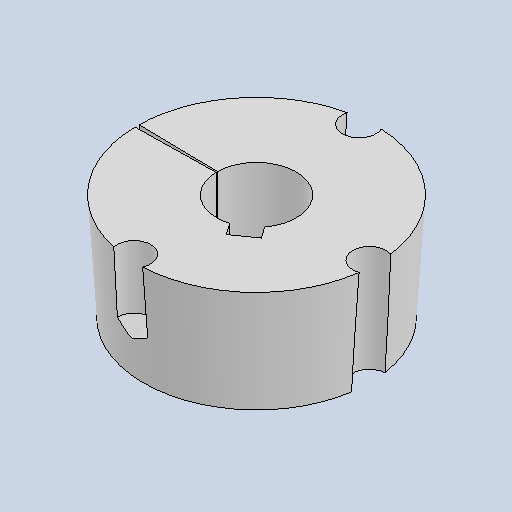
# Autodesk Inventor part: Втулка для шкива
Saved by Autodesk Inventor 2025 (Build 290162010, 162A)
## iProperties
Created: 2024-04-09
Part Number: Втулка для шкива
Material: Generic
Document SubType Name: Modeling
Designer: pokla
Density: 1 g/cm^3
Appearance: Default
Stock Number: Втулка тапербуш
Author: pokla
Autodesk Inventor part; units mm, degrees
ref_plane "YZ Plane" through (0, 0, 0) normal (1, 0, 0) x (0, 1, 0)
ref_plane "XZ Plane" through (0, 0, 0) normal (0, 1, 0) x (-1, 0, 0)
ref_plane "XY Plane" through (0, 0, 0) normal (0, 0, 1) x (1, 0, 0)
sketch "Sketch2" plane through (0, 0, 0) normal (0, 0, 1) x (1, 0, 0)
  line L0 (9.5, 0) -> (9.5, -25.4)
  line L1 (9.5, 0) -> (28.535, 0)
  line L2 (9.5, -25.4) -> (26.985, -25.4)
  line L3 (28.535, 0) -> (26.985, -25.4)
  line L4 (0, -30.48) -> (0, 5.08) projected
  point P0 (0, 0)
  dimension "d5" = 9.5
  dimension "d6" = 25.4
  dimension "d7" = 19.035
  dimension "d8" = 17.485
  constraints: 8 end point, 2 horizontal, 1 horizontal alignment, 1 vertical
  measures "d5" distance from line of point (0, 0) L0
  measures "d6" distance of L0.start L0.end
  measures "d7" distance of L0.start L1.end
  measures "d8" distance of L0.end L2.end
revolve "Revolution1" add sketch "Sketch2" angle 358 mid plane about axis through (0, -10, 0) along (0, 1, 0)
sketch "Sketch3" plane through (0, 0, 0) normal (0, 1, 0) x (-1, 0, 0)
  line L0 (0, 0) -> (-7.055, 10.0756) construction
  line L1 (0, 0) -> (-9.5, 0) construction
  arc A0 (9.4986, 0.1658) -> (9.4986, -0.1658) centre (0, 0) ccw projected
  line L2 (-9.5124, 8.3548) -> (-4.5975, 11.7963)
  line L3 (-9.5124, 8.3548) -> (-7.6276, 5.663)
  line L4 (-4.5975, 11.7963) -> (-2.7127, 9.1045)
  dimension "d10" = 55
  dimension "d11" = 12.3
  dimension "d12" = 6
  constraints: 10 end point, 3 perpendicular, 3 point on circle, 1 horizontal, 1 midpoint
  measures "d10" angle of L1 L0
  measures "d11" distance of L0.end L0.start
  measures "d12" distance of L2.start L2.end
extrude "Extrusion2" cut sketch "Sketch3" against normal through all
sketch "Sketch4" plane through (0, 0, 0) normal (0, 1, 0) x (-1, 0, 0)
  arc A0 (26.9809, 0.471) -> (26.9809, -0.471) centre (0, 0) ccw projected
  point P0 (0, 0)
  point P1 (-26.985, 0)
  constraints: 1 point on circle
sketch "Sketch5" plane through (0, 0, 0) normal (0, 1, 0) x (-1, 0, 0)
  arc A0 (26.9809, 0.471) -> (26.9809, -0.471) centre (0, 0) ccw projected
  arc A1 (26.9809, 0.471) -> (26.9809, -0.471) centre (0, 0) ccw projected
  line L0 (0, 0) -> (26.985, 0) construction
  line L1 (0, 0) -> (3.6164, 41.3358) construction
  line L2 (0, 0) -> (3.8154, -43.6107) construction
  point P0 (0, 0)
  point P1 (-26.6885, 3.989)
  point P2 (-26.6885, -3.989)
  point P3 (2.3519, -26.8823)
  point P4 (2.3519, 26.8823)
  dimension "d18" = 85
  dimension "d21" = 85
  constraints: 6 end point, 2 point on circle, 2 point on line, 1 horizontal
  measures "d18" angle of L0 L1
  measures "d21" angle of L0 L2
hole "Hole1" at (26.985, 0, 0) direction (0, -1, 0) diameter 8 end through all
hole "Hole2" at (-2.3519, 0, -26.8823) at (-2.3519, 0, 26.8823) direction (0, -1, 0) diameter 8 depth 15 tip angle 118
equation "\"d21\" = d18"
body "Solid2"
